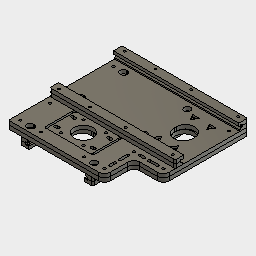
x_carriage humphrito (Autodesk Fusion 360 design; units mm, degrees)
Autodesk Fusion 360 part; units mm, degrees
note: some values were not read from the file. Chosen so that the rebuilt part matches the saved one: how an offset face is resized. Set by a fixed rule: which sketch regions a step uses.
sketch "Sketch1" plane through (0, 0, 0) normal (1, 0, 0) x (0, 0, -1)
  line L0 (0, 0) -> (-127, 0)
  line L1 (-127, 0) -> (-127, 8) construction
  line L2 (-127, 8) -> (0, 8)
  line L3 (0, 8) -> (0, 0)
  line L4 (-127, 4) -> (-123, 0)
  line L5 (-4, 0) -> (0, 4)
  line L6 (-139.5, 14) -> (-121.5, 14)
  line L7 (-121.5, 14) -> (-121.5, -2) construction
  line L8 (-121.5, -2) -> (-139.5, -2)
  line L9 (-139.5, -2) -> (-139.5, 14)
  line L10 (-139.5, 6) -> (-121.5, 6) construction
  line L11 (-128.5, 8.5) -> (-125.5, 8.5)
  line L12 (-125.5, 8.5) -> (-125.5, 3.4142) construction
  line L13 (-125.5, 3.4142) -> (-128.5, 3.4142) construction
  line L14 (-128.5, 3.4142) -> (-128.5, 8.5)
  line L15 (-126.4142, 3.4142) -> (-123.5858, 0.5858)
  line L16 (-125.5, 8.5) -> (-125.5, 8)
  line L17 (-128.5, 3.4142) -> (-126.4142, 3.4142)
  line L18 (-123.5858, 0.5858) -> (-123.5858, -2)
  line L19 (-121.5, 14) -> (-121.5, 8)
  line L20 (-128.5, 6) -> (-139.5, 6)
  line L21 (-127, 4) -> (-127, 8)
  line L22 (-134, 14) -> (-134, -2) construction
  line L23 (-63.5, 8) -> (-63.5, 0) construction
  line L24 (12.5, -2) -> (12.5, 14)
  line L25 (12.5, 14) -> (-5.5, 14)
  line L26 (-5.5, 14) -> (-5.5, -2) construction
  line L27 (-5.5, -2) -> (12.5, -2)
  line L28 (-139.5, -2) -> (12.5, -2)
  line L29 (12.5, -2) -> (12.5, -10)
  line L30 (12.5, -10) -> (-139.5, -10)
  line L31 (-139.5, -10) -> (-139.5, -2)
  line L32 (-76.5, 0) -> (-52, 0)
  line L33 (-52, 0) -> (-52, 4)
  line L34 (-52, 4) -> (-76.5, 4)
  line L35 (-76.5, 4) -> (-76.5, 0)
  line L36 (12.5, -10) -> (-139.5, -10)
  line L37 (-201.5, -18) -> (12.5, -18)
  line L38 (12.5, -18) -> (12.5, -10)
  line L39 (-201.5, -10) -> (-139.5, -10)
  line L40 (-139.5, -10) -> (-139.5, -2)
  line L41 (-139.5, -2) -> (-201.5, -2)
  line L42 (-201.5, -2) -> (-201.5, -10)
  line L43 (-139.5, -10) -> (-201.5, -10)
  line L44 (-201.5, -10) -> (-201.5, -18)
  point P0 (-125, 2)
  dimension "d3" = 8
  dimension "d4" = 127
  dimension "d5" = 45
  dimension "d6" = 4
  dimension "d7" = 45
  dimension "d8" = 4
  dimension "d9" = 18
  dimension "d10" = 4
  dimension "d11" = 3
  dimension "d12" = 0.5
  dimension "d13" = 1.5
  dimension "d14" = 4
  dimension "d15" = 8
  dimension "d16" = 11
  dimension "d17" = 6
  dimension "d19" = 12.5
  dimension "d20" = 8
  dimension "d21" = 4
  dimension "d22" = 24.5
  dimension "d23" = 75
  dimension "d24" = 8
  dimension "d26" = 62
  dimension "d28" = 8
  dimension "d55" = 87.5
  dimension "d230" = 0
  dimension "d231" = 0
  dimension "d232" = 0
  dimension "d233" = 0
  dimension "d252" = 0
  dimension "d253" = 0
  dimension "d254" = 0
  dimension "d255" = 0
  measures "d3" distance of L0.start L2.end
  measures "d4" distance of L1.end L2.end
  measures "d5" angle of L0 L5
  measures "d6" distance of L5.start L5.end
  measures "d7" angle of L0 L4
  measures "d8" distance of L1.end L4.start
  measures "d9" distance of L6.start L6.end
  measures "d10" distance of L7 L12
  measures "d11" distance of L11.start L11.end
  measures "d12" distance of L2 L11
  measures "d13" distance of L1 L14
  measures "d14" distance of L15.start L15.end
  measures "d15" distance of L6 L10
  measures "d16" distance of L9 L14
  measures "d17" distance of L2 L6
  measures "d19" distance of L9 L21
  measures "d20" distance of L24.start L29.end
  measures "d21" distance of L32.start L34.end
  measures "d22" distance of L33.end L34.end
  measures "d23" distance of L21 L33
  measures "d24" distance of L30.end L37.start
  measures "d26" distance of L8.end L41.end
  measures "d28" distance of L39.start L41.end
  measures "d55" distance of L9 L33.end
sketch "Sketch2" plane through (0, 0, 0) normal (0, 1, 0) x (1, 0, 0)
  line L0 (0, -139.5) -> (0, 12.5) construction
  line L1 (0, 12.5) -> (214, 12.5)
  line L2 (214, -139.5) -> (0, -139.5) construction
  line L3 (0, -139.5) -> (0, 12.5)
  line L4 (0, 12.5) -> (152, 12.5)
  line L5 (152, 12.5) -> (152, -201.5) construction
  line L6 (0, -76.5) -> (214, -76.5) construction
  line L7 (214, -76.5) -> (214, -52)
  line L8 (214, -52) -> (0, -52) construction
  line L9 (0, -52) -> (0, -76.5)
  line L10 (152, -64.25) -> (214, -64.25) construction
  line L11 (64.5, -201.5) -> (89, -201.5)
  line L12 (89, -201.5) -> (89, 12.5) construction
  line L13 (89, 12.5) -> (64.5, 12.5)
  line L14 (64.5, 12.5) -> (64.5, -201.5) construction
  line L15 (0, -76.5) -> (0, -52)
  line L16 (0, -76.5) -> (0, -52)
  line L17 (76.75, -201.5) -> (76.75, -139.5) construction
  line L18 (29.75, -139.5) -> (123.75, -139.5)
  line L19 (123.75, -139.5) -> (123.75, -201.5)
  line L20 (123.75, -201.5) -> (29.75, -201.5)
  line L21 (29.75, -201.5) -> (29.75, -139.5)
  circle A0 centre (76.75, -170.5) radius 19.5
  line L22 (123.75, -201.5) -> (29.75, -139.5) construction
  circle A1 centre (53.18, -194.07) radius 2.5
  line L23 (53.18, -194.07) -> (100.32, -194.07) construction
  line L24 (100.32, -194.07) -> (100.32, -146.93) construction
  line L25 (100.32, -146.93) -> (53.18, -146.93) construction
  line L26 (53.18, -146.93) -> (53.18, -194.07) construction
  circle A2 centre (100.32, -194.07) radius 2.5
  circle A3 centre (100.32, -146.93) radius 2.5
  circle A4 centre (53.18, -146.93) radius 2.5
  line L27 (53.18, -194.07) -> (100.32, -146.93) construction
  line L28 (79, -151) -> (74.5, -151)
  arc A5 (74.5, -151) -> (74.5, -190) centre (74.5, -170.5) ccw
  line L29 (74.5, -190) -> (79, -190)
  arc A6 (79, -190) -> (79, -151) centre (79, -170.5) ccw
  line L30 (79, -170.5) -> (74.5, -170.5) construction
  line L31 (0, -201.5) -> (152, -201.5)
  line L32 (214, 12.5) -> (214, -139.5)
  line L33 (53.18, -194.07) -> (29.75, -194.07) construction
  line L34 (0, -139.5) -> (0, -201.5)
  line L35 (0, -201.5) -> (0, 12.5)
  line L36 (0, 0) -> (0, -127)
  line L37 (0, -52) -> (0, -139.5)
  line L38 (0, -139.5) -> (0, -52)
  line L39 (152, -201.5) -> (64.5, -201.5)
  line L40 (0, 12.5) -> (-25, 12.5)
  line L41 (-25, 12.5) -> (-25, -201.5)
  line L42 (-25, -201.5) -> (0, -201.5) construction
  line L43 (0, -201.5) -> (0, 12.5) construction
  line L44 (0, -201.5) -> (152, -201.5) construction
  line L45 (214, -139.5) -> (152, -139.5)
  line L46 (152, -139.5) -> (152, -201.5)
  line L47 (152, -201.5) -> (214, -201.5)
  line L48 (214, -201.5) -> (214, -139.5)
  line L49 (0, -5.5) -> (214, -5.5) construction
  line L50 (0, -121.5) -> (214, -121.5) construction
  line L51 (18, 12.5) -> (18, -201.5) construction
  line L52 (214, 12.5) -> (214, -5.5)
  line L53 (134, 12.5) -> (134, -201.5) construction
  circle A7 centre (183, -64.25) radius 19.5 construction
  line L54 (18, -201.5) -> (0, -201.5)
  line L55 (18, 30.7845) -> (134, 30.7845)
  line L56 (76, 30.7845) -> (76, 24.5879) construction
  line L57 (38.75, -188) -> (114.75, -188) construction
  line L58 (114.75, -188) -> (114.75, -153) construction
  line L59 (114.75, -153) -> (38.75, -153) construction
  line L60 (38.75, -153) -> (38.75, -188) construction
  line L61 (38.75, -188) -> (114.75, -153) construction
  line L62 (114.75, -188) -> (38.75, -153) construction
  circle A8 centre (38.75, -153) radius 2.5
  circle A9 centre (38.75, -188) radius 2.5
  circle A10 centre (114.75, -153) radius 2.5
  circle A11 centre (114.75, -188) radius 2.5
  line L63 (34.75, -159.9282) -> (46.75, -153)
  line L64 (46.75, -153) -> (34.75, -146.0718)
  line L65 (34.75, -146.0718) -> (34.75, -159.9282)
  line L66 (38.75, -148.3812) -> (34.75, -150.6906) construction
  line L67 (34.75, -150.6906) -> (34.75, -155.3094)
  line L68 (34.75, -155.3094) -> (38.75, -157.6188) construction
  line L69 (38.75, -157.6188) -> (42.75, -155.3094)
  line L70 (42.75, -155.3094) -> (42.75, -150.6906) construction
  line L71 (42.75, -150.6906) -> (38.75, -148.3812)
  line L72 (34.75, -181.0718) -> (34.75, -194.9282)
  line L73 (34.75, -194.9282) -> (46.75, -188)
  line L74 (46.75, -188) -> (34.75, -181.0718)
  line L75 (118.75, -159.9282) -> (106.75, -153)
  line L76 (118.75, -146.0718) -> (118.75, -159.9282)
  line L77 (106.75, -153) -> (118.75, -146.0718)
  line L78 (106.75, -188) -> (118.75, -181.0718)
  line L79 (118.75, -181.0718) -> (118.75, -194.9282)
  line L80 (118.75, -194.9282) -> (106.75, -188)
  line L81 (214, -201.5) -> (-25, -201.5)
  line L82 (-25, -201.5) -> (-25, -226.5)
  line L83 (-25, -226.5) -> (214, -226.5)
  line L84 (214, -226.5) -> (214, -201.5)
  line L85 (214, 12.5) -> (239, 12.5)
  line L86 (239, 12.5) -> (239, -226.5)
  line L87 (239, -226.5) -> (214, -226.5)
  line L88 (214, -226.5) -> (214, 12.5)
  line L89 (0, -201.5) -> (0, -226.5)
  circle A12 centre (38.75, -153) radius 6.25
  line L90 (48.75, -142.5) -> (104.75, -142.5) construction
  line L91 (104.75, -142.5) -> (104.75, -198.5) construction
  line L92 (104.75, -198.5) -> (48.75, -198.5) construction
  line L93 (48.75, -198.5) -> (48.75, -142.5) construction
  line L94 (48.75, -142.5) -> (104.75, -198.5) construction
  line L95 (104.75, -142.5) -> (48.75, -198.5) construction
  point P0 (0, -201.5)
  point P1 (0, -139.5)
  point P2 (0, -52)
  point P3 (0, -76.5)
  point P4 (76.75, -170.5)
  point P5 (53.18, -194.07)
  point P6 (0, -201.5)
  point P7 (0, -121.5)
  point P8 (0, -5.5)
  point P9 (183, -64.25)
  point P10 (76.75, -170.5)
  point P11 (38.75, -153)
  point P12 (38.75, -153)
  point P13 (38.75, -188)
  point P14 (76.75, -170.5)
  dimension "d34" = 94
  dimension "d36" = 39
  dimension "d37" = 5
  dimension "d38" = 47.14
  dimension "d39" = 4.5
  dimension "d40" = 19.5
  dimension "d56" = 25
  dimension "d63" = 18
  dimension "d112" = 18
  dimension "d209" = 18
  dimension "d272" = 35
  dimension "d273" = 76
  dimension "d274" = 5
  dimension "d275" = 8
  dimension "d282" = 25
  dimension "d283" = 25
  dimension "d298" = 12.5
  dimension "d299" = 56
  measures "d34" distance of L19.end L20.end
  measures "d36" diameter of A0
  measures "d37" diameter of A1
  measures "d38" distance of P5 L23.end
  measures "d39" distance of A6.centre A5.centre
  measures "d40" radius of A6
  measures "d56" distance of L0.end L40.end
  measures "d63" distance of L1 L49
  measures "d112" distance of L35 L51
  measures "d209" distance of L5 L53
  measures "d272" distance of L57.end L58.end
  measures "d273" distance of L58.end P12
  measures "d274" diameter of A8
  measures "d275" distance of L68 L71
  measures "d282" distance of L41.end L82.end
  measures "d283" distance of L83.end L86.end
  measures "d298" diameter of A12
  measures "d299" distance of L90.start L90.end
sketch "Sketch3" plane through (0, 0, 0) normal (0, 1, 0) x (1, 0, 0)
  line L0 (-25, 12.5) -> (-25, -201.5)
  line L1 (0, -5.5) -> (214, -5.5)
  line L2 (0, 12.5) -> (214, 12.5)
  line L3 (0, 12.5) -> (-25, 12.5)
  line L4 (0, -5.5) -> (-25, -5.5)
  line L5 (214, 12.5) -> (214, -5.5)
  line L6 (239, 5.5) -> (-25, 5.5) construction
  circle A0 centre (-12.5, 5.5) radius 2.25
  circle A1 centre (-12.5, 5.5) radius 2.5
  line L7 (-9.75, 4.5) -> (-9.75, 6.5)
  arc A2 (-9.75, 6.5) -> (-15.25, 6.5) centre (-12.5, 6.5) ccw
  line L8 (-15.25, 6.5) -> (-15.25, 4.5)
  arc A3 (-15.25, 4.5) -> (-9.75, 4.5) centre (-12.5, 4.5) ccw
  line L9 (-12.5, 4.5) -> (-12.5, 6.5) construction
  circle A4 centre (-12.5, 5.5) radius 6.25 construction
  line L10 (107, 5.5) -> (107, 12.5) construction
  circle A5 centre (226.5, 5.5) radius 2.5
  circle A6 centre (226.5, 5.5) radius 2.25
  circle A7 centre (226.5, 5.5) radius 6.25 construction
  line L11 (223.75, 4.5) -> (223.75, 6.5)
  arc A8 (223.75, 4.5) -> (229.25, 4.5) centre (226.5, 4.5) ccw
  line L12 (226.5, 4.5) -> (226.5, 6.5) construction
  line L13 (229.25, 6.5) -> (229.25, 4.5)
  arc A9 (229.25, 6.5) -> (223.75, 6.5) centre (226.5, 6.5) ccw
  circle A10 centre (52.5, 5.5) radius 2.25
  arc A11 (55.25, 6.5) -> (49.75, 6.5) centre (52.5, 6.5) ccw
  arc A12 (49.75, 4.5) -> (55.25, 4.5) centre (52.5, 4.5) ccw
  circle A13 centre (52.5, 5.5) radius 2.5
  line L14 (52.5, 4.5) -> (52.5, 6.5) construction
  line L15 (55.25, 4.5) -> (55.25, 6.5)
  circle A14 centre (52.5, 5.5) radius 6.25 construction
  line L16 (49.75, 6.5) -> (49.75, 4.5)
  circle A15 centre (127.5, 5.5) radius 2.25
  arc A16 (124.75, 4.5) -> (130.25, 4.5) centre (127.5, 4.5) ccw
  circle A17 centre (127.5, 5.5) radius 2.5
  line L17 (124.75, 6.5) -> (124.75, 4.5)
  arc A18 (130.25, 6.5) -> (124.75, 6.5) centre (127.5, 6.5) ccw
  line L18 (127.5, 4.5) -> (127.5, 6.5) construction
  line L19 (130.25, 4.5) -> (130.25, 6.5)
  circle A19 centre (127.5, 5.5) radius 6.25 construction
  line L20 (-41.6156, -63.5) -> (240.5702, -63.5) construction
  line L21 (240.5702, -5.5) -> (240.5702, -121.5) construction
  line L22 (0, -121.5) -> (214, -121.5)
  circle A20 centre (-12.5, -132.5) radius 2.5
  circle A21 centre (52.5, -132.5) radius 2.5
  circle A22 centre (127.5, -132.5) radius 2.5
  circle A23 centre (226.5, -132.5) radius 2.5
  circle A24 centre (-12.5, -132.5) radius 2.25
  circle A25 centre (52.5, -132.5) radius 2.25
  circle A26 centre (127.5, -132.5) radius 2.25
  circle A27 centre (226.5, -132.5) radius 2.25
  line L23 (-12.5, 4.5) -> (-12.5, 4.3)
  arc A28 (-5.75, 6.5) -> (-19.25, 6.5) centre (-12.5, 6.5) ccw construction
  line L24 (-19.25, 6.5) -> (-19.25, 4.5)
  arc A29 (-19.25, 4.5) -> (-5.75, 4.5) centre (-12.5, 4.5) ccw
  line L25 (-5.75, 4.5) -> (-5.75, 6.5)
  line L26 (-19.25, 12.5) -> (-5.75, 12.5)
  line L27 (-5.75, 12.5) -> (-5.75, 6.5)
  line L28 (-5.75, 6.5) -> (-19.25, 6.5) construction
  line L29 (-19.25, 6.5) -> (-19.25, 12.5)
  arc A30 (59.25, 6.5) -> (45.75, 6.5) centre (52.5, 6.5) ccw construction
  line L30 (45.75, 6.5) -> (45.75, 4.5)
  arc A31 (45.75, 4.5) -> (59.25, 4.5) centre (52.5, 4.5) ccw
  line L31 (59.25, 4.5) -> (59.25, 6.5)
  arc A32 (134.25, 6.5) -> (120.75, 6.5) centre (127.5, 6.5) ccw construction
  line L32 (120.75, 6.5) -> (120.75, 4.5)
  arc A33 (120.75, 4.5) -> (134.25, 4.5) centre (127.5, 4.5) ccw
  line L33 (134.25, 4.5) -> (134.25, 6.5)
  line L34 (233.25, 6.5) -> (233.25, 4.5)
  arc A34 (219.75, 4.5) -> (233.25, 4.5) centre (226.5, 4.5) ccw
  line L35 (219.75, 4.5) -> (219.75, 6.5)
  arc A35 (233.25, 6.5) -> (219.75, 6.5) centre (226.5, 6.5) ccw construction
  line L36 (219.75, 12.5) -> (233.25, 12.5)
  line L37 (233.25, 12.5) -> (233.25, 6.5)
  line L38 (233.25, 6.5) -> (219.75, 6.5) construction
  line L39 (219.75, 6.5) -> (219.75, 12.5)
  line L40 (120.75, 12.5) -> (134.25, 12.5)
  line L41 (134.25, 12.5) -> (134.25, 6.5)
  line L42 (134.25, 6.5) -> (120.75, 6.5) construction
  line L43 (120.75, 6.5) -> (120.75, 12.5)
  line L44 (45.75, 12.5) -> (59.25, 12.5)
  line L45 (59.25, 12.5) -> (59.25, 6.5)
  line L46 (59.25, 6.5) -> (45.75, 6.5) construction
  line L47 (45.75, 6.5) -> (45.75, 12.5)
  circle A36 centre (-12.5, -132.5) radius 6.75
  circle A37 centre (52.5, -132.5) radius 6.75
  circle A38 centre (127.5, -132.5) radius 6.75
  circle A39 centre (226.5, -132.5) radius 6.75
  line L48 (239, 12.5) -> (239, -226.5)
  point P0 (-12.5, 5.5)
  point P1 (226.5, 5.5)
  point P2 (52.5, 5.5)
  point P3 (127.5, 5.5)
  dimension "d84" = 4.5
  dimension "d85" = 5
  dimension "d86" = 2.75
  dimension "d87" = 2
  dimension "d88" = 12.5
  dimension "d89" = 12.5
  dimension "d92" = -65
  dimension "d93" = 0
  dimension "d96" = -140
  dimension "d97" = 0
  dimension "d98" = 55
  dimension "d99" = 85
  dimension "d100" = 74
  dimension "d199" = 7
  dimension "d202" = 4.5
  dimension "d242" = 0.2
  dimension "d243" = 4
  dimension "d244" = 6.75
  dimension "d245" = 4
  dimension "d246" = 4
  dimension "d247" = 4
  dimension "d271" = 13.5
  dimension "d284" = 12.5
  measures "d84" diameter of A0
  measures "d85" diameter of A1
  measures "d86" radius of A2
  measures "d87" distance of A3.centre A2.centre
  measures "d88" distance of L0 P0
  measures "d89" diameter of A4
  measures "d199" distance of L2.end L6
  measures "d202" diameter of A24
  measures "d242" distance of A3.centre L23.end
  measures "d244" radius of A29
  measures "d271" diameter of A36
  measures "d284" distance of P1 L48
sketch "Sketch4" plane through (0, 0, 0) normal (0, 1, 0) x (1, 0, 0)
  line L0 (0, 12.5) -> (-25, 12.5) construction
  line L1 (-12.5, 12.5) -> (-12.5, -201.5) construction
  line L2 (-25, -214) -> (214, -214) construction
  line L3 (214, -201.5) -> (214, -139.5) construction
  circle A0 centre (-12.5, -18) radius 2.5
  circle A1 centre (-12.5, -214) radius 2.5
  circle A2 centre (164.5, -214) radius 2.5
  line L4 (164.5, -214) -> (164.5, 12.5) construction
  line L5 (0, 12.5) -> (164.5, 12.5) construction
  line L6 (-12.5, 12.5) -> (0, 12.5) construction
  line L7 (0, -5.5) -> (-25, -5.5) construction
  line L8 (-12.5, -18) -> (14.3422, -18) construction
  line L9 (0, -5.5) -> (164.5, -5.5) construction
  line L10 (164.5, -5.5) -> (164.5, -12) construction
  line L11 (14.3422, -18) -> (158.5, -18) construction
  circle A3 centre (-12.5, -109) radius 2.5
  line L12 (-12.5, -109) -> (158.5, -109) construction
  line L13 (0, -121.5) -> (214, -121.5) construction
  line L14 (0, -121.5) -> (-12.5, -121.5) construction
  line L15 (-12.5, -121.5) -> (-12.5, -109) construction
  line L16 (214, -111.25) -> (152, -111.25)
  line L17 (152, -111.25) -> (152, -17.25)
  line L18 (152, -17.25) -> (214, -17.25)
  line L19 (214, -17.25) -> (214, -111.25)
  line L20 (214, -111.25) -> (152, -17.25) construction
  line L21 (152, -111.25) -> (214, -17.25) construction
  line L22 (123.75, -139.5) -> (123.75, -201.5) construction
  line L23 (123.75, -201.5) -> (29.75, -201.5) construction
  line L24 (152, -139.5) -> (152, -201.5) construction
  line L25 (214, -139.5) -> (0, -139.5) construction
  line L26 (-25, 12.5) -> (-25, -201.5) construction
  line L27 (0, -139.5) -> (-25, -139.5) construction
  line L28 (-12.5, -121.5) -> (-25, -121.5) construction
  circle A4 centre (-12.5, -152) radius 2.5
  line L29 (-12.5, -152) -> (-12.5, -139.5)
  circle A5 centre (164.5, -152) radius 2.5
  line L30 (-12.5, -152) -> (164.5, -152) construction
  line L31 (0, -5.5) -> (214, -5.5) construction
  circle A6 centre (226.5, -114.25) radius 2.5
  circle A7 centre (226.5, -14.25) radius 2.5
  line L32 (-25, -201.5) -> (0, -201.5) construction
  line L33 (163.5, -62) -> (163.5, -66.5)
  arc A8 (163.5, -66.5) -> (202.5, -66.5) centre (183, -66.5) ccw
  line L34 (202.5, -66.5) -> (202.5, -62)
  arc A9 (202.5, -62) -> (163.5, -62) centre (183, -62) ccw
  line L35 (183, -62) -> (183, -66.5) construction
  circle A10 centre (226.5, -14.25) radius 6.25 construction
  circle A11 centre (226.5, -114.25) radius 6.25 construction
  line L36 (226.5, -114.25) -> (226.5, -14.25) construction
  line L37 (183, -64.25) -> (226.5, -64.25) construction
  line L38 (239, 12.5) -> (239, -226.5)
  line L39 (214, -5.5) -> (239, -5.5) construction
  line L40 (226.5, -5.5) -> (226.5, -14.25) construction
  line L41 (214, -201.5) -> (-25, -201.5)
  circle A12 centre (30.5, -214) radius 2.5
  circle A13 centre (121.5, -214) radius 2.5
  line L42 (18, 12.5) -> (18, -201.5)
  line L43 (134, 12.5) -> (134, -201.5)
  line L44 (164.5, -152) -> (167, -152)
  line L45 (164.5, -152) -> (226.5, -152) construction
  circle A14 centre (226.5, -152) radius 2.5
  line L46 (226.5, -152) -> (226.5, -114.25) construction
  point P0 (183, -64.25)
  point P1 (183, -64.25)
  point P2 (214, -201.5)
  point P3 (183, -64.25)
  dimension "d101" = 5
  dimension "d102" = 105
  dimension "d103" = 91
  dimension "d104" = 12.5
  dimension "d105" = 12.5
  dimension "d117" = 19.5
  dimension "d118" = 4.5
  dimension "d213" = 12.5
  dimension "d327" = 100
  dimension "d355" = 12.5
  dimension "d356" = 12.5
  dimension "d357" = 12.5
  measures "d101" diameter of A1
  measures "d102" distance of A1.centre A3.centre
  measures "d103" distance of A0.centre A3.centre
  measures "d104" distance of L7 A0.centre
  measures "d105" distance of A2.centre L24
  measures "d117" radius of A8
  measures "d118" distance of A9.centre A8.centre
  measures "d213" diameter of A10
  measures "d327" distance of A6.centre A7.centre
  measures "d355" distance of A1.centre L41
  measures "d356" distance of A12.centre L42
  measures "d357" distance of A13.centre L43
sketch "Sketch6" plane through (0, 0, 0) normal (0, 1, 0) x (1, 0, 0)
  line L0 (-25, 12.5) -> (239, 12.5)
  line L1 (239, 12.5) -> (239, -226.5)
  line L2 (239, -226.5) -> (-25, -226.5)
  line L3 (-25, -226.5) -> (-25, 12.5)
  point P0 (-25, 12.5)
  point P1 (214, -201.5)
  point P2 (239, -226.5)
extrude "Extrude2" add sketch "Sketch6" against normal up to surface (8 mm away) from surface at -2 makes body 1
extrude "Extrude3" cut sketch "Sketch2" sketch "Sketch4" along normal up to surface contours A0 | A0 L28 L29 A6 | A0 L28 A5 L29 of sketch 2 contours L33 A8 L34 A9 start surface through (0, -2, -12.5) normal (0, 1, 0) end surface through (0, -10, -12.5) normal (0, 1, 0) offset 0 bodies 1
extrude "Extrude4" cut sketch "Sketch4" against normal up to surface (8 mm away) from surface at -2 contours A0 | A1 | A2 | A3 | A4 | A5 | A6 | A7 | A12 | A13 | A14 bodies 1
extrude "Extrude5" cut sketch "Sketch3" against normal up to surface (8 mm away) from surface at -2 contours A0 | A1 | L7 A2 L8 A3 | A5 | A6 | L11 A8 L13 A9 | A10 | A11 A12 L15 L16 | A13 | A15 | A16 L17 A18 L19 | A17 bodies 1
extrude "Extrude6" cut sketch "Sketch3" against normal up to surface (8 mm away) from surface at -2 contours A20 | A21 | A22 | A23 | A24 | A25 | A26 | A27 bodies 1
sketch "Sketch8" plane through (0, 0, 0) normal (0, 1, 0) x (1, 0, 0)
  line L0 (18, 12.5) -> (18, -201.5) construction
  line L1 (0, -201.5) -> (0, 12.5) construction
  line L2 (134, 12.5) -> (134, -201.5) construction
  line L3 (0, -201.5) -> (18, -201.5) construction
  line L4 (18, -201.5) -> (134, -201.5) construction
  line L5 (76, -201.5) -> (76, -159.0464) construction
  circle A0 centre (9, -214) radius 6.5 construction
  line L6 (9, -201.5) -> (9, -214) construction
  circle A1 centre (9, -214) radius 2.5
  circle A2 centre (9, -214) radius 2.25
  line L7 (8, -216.75) -> (10, -216.75)
  arc A3 (10, -216.75) -> (10, -211.25) centre (10, -214) ccw
  line L8 (10, -211.25) -> (8, -211.25)
  arc A4 (8, -211.25) -> (8, -216.75) centre (8, -214) ccw
  line L9 (8, -214) -> (10, -214) construction
  arc A5 (8, -106.25) -> (8, -111.75) centre (8, -109) ccw
  arc A6 (10, -111.75) -> (10, -106.25) centre (10, -109) ccw
  line L10 (8, -109) -> (10, -109) construction
  line L11 (10, -106.25) -> (8, -106.25)
  circle A7 centre (9, -109) radius 6.5 construction
  line L12 (8, -111.75) -> (10, -111.75)
  circle A8 centre (9, -109) radius 2.25
  circle A9 centre (9, -109) radius 2.5
  line L13 (9, -214) -> (9, -109) construction
  line L14 (9, -109) -> (9, -18) construction
  arc A10 (8, -15.25) -> (8, -20.75) centre (8, -18) ccw
  arc A11 (10, -20.75) -> (10, -15.25) centre (10, -18) ccw
  line L15 (8, -18) -> (10, -18) construction
  line L16 (10, -15.25) -> (8, -15.25)
  circle A12 centre (9, -18) radius 6.25 construction
  line L17 (8, -20.75) -> (10, -20.75)
  circle A13 centre (9, -18) radius 2.25
  circle A14 centre (9, -18) radius 2.5
  line L18 (0, -121.5) -> (214, -121.5)
  line L19 (0, -5.5) -> (164.5, -5.5) construction
  circle A15 centre (143, -214) radius 2.5
  circle A16 centre (143, -109) radius 2.5
  circle A17 centre (143, -18) radius 2.5
  circle A18 centre (143, -18) radius 2.25
  circle A19 centre (143, -109) radius 2.25
  circle A20 centre (143, -214) radius 2.25
  arc A21 (8, -11.25) -> (8, -24.75) centre (8, -18) ccw
  line L20 (8, -24.75) -> (10, -24.75)
  arc A22 (10, -24.75) -> (10, -11.25) centre (10, -18) ccw
  line L21 (10, -11.25) -> (8, -11.25)
  arc A23 (8, -102.25) -> (8, -115.75) centre (8, -109) ccw
  line L22 (8, -115.75) -> (10, -115.75)
  arc A24 (10, -115.75) -> (10, -102.25) centre (10, -109) ccw
  line L23 (10, -102.25) -> (8, -102.25)
  arc A25 (8, -207.25) -> (8, -220.75) centre (8, -214) ccw
  line L24 (8, -220.75) -> (10, -220.75)
  arc A26 (10, -220.75) -> (10, -207.25) centre (10, -214) ccw
  line L25 (10, -207.25) -> (8, -207.25)
  circle A27 centre (143, -18) radius 6.75
  circle A28 centre (143, -109) radius 6.75
  circle A29 centre (143, -214) radius 6.75
  line L26 (-25, -226.5) -> (214, -226.5)
  point P0 (9, -214)
  point P1 (9, -109)
  point P2 (9, -109)
  point P3 (9, -18)
  point P4 (9, -18)
  dimension "d129" = 13
  dimension "d131" = 5
  dimension "d132" = 4.5
  dimension "d133" = 2.75
  dimension "d134" = 2
  dimension "d135" = 13
  dimension "d136" = 5
  dimension "d137" = 4.5
  dimension "d138" = 2.75
  dimension "d139" = 2
  dimension "d140" = 12.5
  dimension "d141" = 5
  dimension "d142" = 4.5
  dimension "d143" = 2.75
  dimension "d144" = 2
  dimension "d146" = 12.5
  dimension "d148" = 171
  dimension "d212" = 4.5
  dimension "d264" = 4
  dimension "d265" = 4
  dimension "d266" = 4
  dimension "d267" = 13.5
  dimension "d285" = 12.5
  dimension "d286" = 12.5
  measures "d129" diameter of A0
  measures "d131" diameter of A1
  measures "d132" diameter of A2
  measures "d133" radius of A3
  measures "d134" distance of A4.centre A3.centre
  measures "d135" diameter of A7
  measures "d136" diameter of A9
  measures "d137" diameter of A8
  measures "d138" radius of A6
  measures "d139" distance of A5.centre A6.centre
  measures "d140" diameter of A12
  measures "d141" diameter of A14
  measures "d142" diameter of A13
  measures "d143" radius of A11
  measures "d144" distance of A10.centre A11.centre
  measures "d146" distance of P4 L19
  measures "d212" diameter of A20
  measures "d267" diameter of A27
  measures "d285" distance of P0 L26
  measures "d286" distance of P2 L18
extrude "Extrude7" cut sketch "Sketch8" against normal up to surface (8 mm away) from surface at -2 contours A1 | A2 | L7 A3 L8 A4 | A5 A6 L11 L12 | A8 | A9 | A10 A11 L16 L17 | A13 | A14 | A15 | A16 | A17 | A18 | A19 | A20 bodies 1
extrude "Extrude8" add sketch "Sketch1" along normal up to surface (264 mm away) from surface at -25 separate body contours L4 L8 L9 L14 L15 L17 L18 L20 L28 makes body 2
extrude "Extrude9" add sketch "Sketch1" along normal up to surface (264 mm away) from surface at -25 separate body contours L2 L6 L9 L11 L14 L16 L19 L20 makes body 3
ref_plane "WorkPlane1" through (107, -6, 63.5) normal (0, 0, -1) x (1, 0, 0)
mirror "Mirror1" about plane through (107, -6, 63.5) normal (0, 0, -1) of bodies 2 3 makes body 4 at (151, -2, -1.8905) makes body 5 at (63, 14, -6.5)
copy_body "CopyPasteBodies2" bodies 1 makes body 6
move_body "Move3" bodies 6 to x (1, 0, 0) y (0, 1, 0) z (0, 0, 1) at (0, -8, 0)
copy_body "CopyPasteBodies1" bodies 2 3 makes body 7 makes body 8
move_body "Move1" bodies 7 8 to x (0, 0, -1) y (0, -1, 0) z (-1, 0, 0) at (157.2361, -53.9388, 98.5858)
move_body "Move2" bodies 7 8 to x (1, 0, 0) y (0, 1, 0) z (0, 0, 1) at (-17.7361, 33.9388, 127.9142)
move_face "MoveFace1" by (0, 18, -25) 2 faces at (3.6667, -22.4714, 251.5) (3.6667, -29.5, 251.5) on bodies 7 8
ref_plane "WorkPlane2" through (76, 0, -27.6862) normal (-1, 0, 0) x (0, 0, 1)
mirror "Mirror2" about plane through (76, 0, -27.6862) normal (-1, 0, 0) of bodies 8 7 makes body 9 at (146, -34, 146.8333) makes body 10 at (141.3905, -18, 146.8333)
extrude "Extrude10" cut sketch "Sketch3" along normal up to surface (16 mm away) from surface at -10 contours A0 | A1 | A5 | A6 | A10 | A13 | A15 | A17 | A20 | A21 | A22 | A23 | A24 | A25 | A26 | A27 bodies 2 4
extrude "Extrude11" cut sketch "Sketch3" along normal up to surface (8 mm away) from surface at 6 contours A0 | A6 | A10 | A15 | A24 | A25 | A26 | A27 bodies 3 5
extrude "Extrude19" cut sketch "Sketch8" against normal up to surface (8 mm away) from surface at -18 contours A1 | A2 | A8 | A9 | A13 | A14 | A15 | A16 | A17 | A18 | A19 | A20 bodies 7 10
extrude "Extrude20" cut sketch "Sketch8" against normal up to surface (8 mm away) from surface at -26 contours A2 | A8 | A13 | A18 | A19 | A20 bodies 8 9
sketch "Sketch2 (2)" plane through (0, 0, 0) normal (0, 1, 0) x (1, 0, 0) in component "Glide_screw"
  circle A0 centre (0, 0) radius 2.5
  line L0 (2.3094, 4) -> (-2.3094, 4)
  line L1 (-2.3094, 4) -> (-4.6188, 0)
  line L2 (-4.6188, 0) -> (-2.3094, -4)
  line L3 (-2.3094, -4) -> (2.3094, -4)
  line L4 (2.3094, -4) -> (4.6188, 0)
  line L5 (4.6188, 0) -> (2.3094, 4)
  circle A1 centre (0, 0) radius 6.25
  circle A2 centre (0, 0) radius 2.7
  dimension "d216" = 5
  dimension "d217" = 8
  dimension "d218" = 12.5
  dimension "d219" = 5.4
  dimension "d226" = 0
  dimension "d227" = 0
  dimension "d228" = 0
  dimension "d229" = 0
  dimension "d248" = 0
  dimension "d249" = 0
  dimension "d250" = 0
  dimension "d251" = 0
  measures "d216" diameter of A0
  measures "d217" distance of L0 L3
  measures "d218" diameter of A1
  measures "d219" diameter of A2
extrude "Extrude1" add sketch "Sketch2 (2)" against normal blind 25 separate body contours A0 makes body 11 in component "Glide_screw"
extrude "Extrude2'" add sketch "Sketch2 (2)" along normal blind 3.6 contours A0 | L0 L1 L2 L3 L4 L5 | A2 bodies 11 in component "Glide_screw"
extrude "Extrude3'" add sketch "Sketch2 (2)" against normal blind 1 separate body contours L0 L1 L2 L3 L4 L5 | A1 makes body 12 in component "Glide_screw"
thread "Thread1" "ISO Metric profile 5.0 M5x0.8 6g" major diameter 4.901 minor diameter 3.9895 pitch 0.8 angle 60 resizes the face on face at (2.4876, -8.3333, 0.2489) on bodies 11 in component "Glide_screw"
sketch "Sketch10" plane through (0, 0, 0) normal (0, 1, 0) x (1, 0, 0)
extrude "Extrude12" cut sketch "Sketch3" against normal up to surface (8 mm away) from surface at -10 contours L3 L24 A29 L25 L26 L27 L29 | L2 L30 A31 L31 L44 L45 L47 | L2 L32 A33 L33 L40 L41 L43 | L34 A34 L35 L36 L37 L39 | A36 | A37 | A38 | A39 bodies 6
extrude "Extrude13" cut sketch "Sketch8" along normal up to surface (8 mm away) from surface at -10 contours A21 L20 A22 L21 | A23 L22 A24 L23 | A25 L24 A26 L25 | A27 | A28 | A29 bodies 1
extrude "Extrude14" cut sketch "Sketch2" against normal up to surface (8 mm away) from surface at -10 contours A8 | A9 | A10 | A11 bodies 6
extrude "Extrude15" cut sketch "Sketch2" along normal blind 4 from surface at -18 contours L63 L64 L65 L67 L69 L71 A12 | L63 L65 A12 | L63 L64 A12 | L64 L65 A12 | L72 L73 L74 | L75 L76 L77 | L78 L79 L80 bodies 6
sketch "Sketch11" plane through (0, 0, 0) normal (0, 1, 0) x (1, 0, 0)
  line L0 (29.75, -201.5) -> (29.75, -139.5) construction
  line L1 (123.75, -139.5) -> (123.75, -201.5) construction
  line L2 (214, -139.5) -> (0, -139.5)
  line L3 (214, -201.5) -> (-25, -201.5)
  line L4 (25.75, -139.5) -> (25.75, -201.5)
  line L5 (127.75, -139.5) -> (127.75, -201.5)
  dimension "d287" = 4
  dimension "d288" = 4
  measures "d287" distance of L0 L4
  measures "d288" distance of L1 L5
extrude "Extrude16" cut sketch "Sketch11" against normal up to surface (8 mm away) from surface at -2 bodies 1
sketch "Sketch12" plane through (0, 0, 0) normal (0, 1, 0) x (1, 0, 0)
  line L0 (41.5, -150.25) -> (36, -150.25)
  arc A0 (36, -150.25) -> (36, -155.75) centre (36, -153) ccw
  line L1 (36, -155.75) -> (41.5, -155.75)
  arc A1 (41.5, -155.75) -> (41.5, -150.25) centre (41.5, -153) ccw
  line L2 (41.5, -153) -> (36, -153) construction
  circle A2 centre (36, -153) radius 6.25 construction
  circle A3 centre (41.5, -153) radius 6.25 construction
  curve K0
  line L3 (76.75, -201.5) -> (76.75, -139.5)
  line L4 (112, -150.25) -> (117.5, -150.25)
  line L5 (117.5, -155.75) -> (112, -155.75)
  arc A4 (117.5, -155.75) -> (117.5, -150.25) centre (117.5, -153) ccw
  arc A5 (112, -150.25) -> (112, -155.75) centre (112, -153) ccw
  arc A6 (41.5, -190.75) -> (41.5, -185.25) centre (41.5, -188) ccw
  line L6 (41.5, -190.75) -> (36, -190.75)
  arc A7 (36, -185.25) -> (36, -190.75) centre (36, -188) ccw
  line L7 (36, -185.25) -> (41.5, -185.25)
  line L8 (112, -190.75) -> (117.5, -190.75)
  arc A8 (117.5, -190.75) -> (117.5, -185.25) centre (117.5, -188) ccw
  arc A9 (112, -185.25) -> (112, -190.75) centre (112, -188) ccw
  line L9 (117.5, -185.25) -> (112, -185.25)
  point P0 (38.75, -153)
  point P1 (114.75, -153)
  point P2 (114.75, -188)
  point P3 (38.75, -188)
  point P4 (38.75, -153)
  dimension "d340" = 5.5
  dimension "d341" = 2.75
  dimension "d342" = 12.5
  measures "d340" distance of A1.centre A0.centre
  measures "d341" radius of A1
  measures "d342" diameter of A3
sketch "Sketch14" plane through (0, 0, 0) normal (0, 1, 0) x (1, 0, 0)
  line L0 (53.18, -194.07) -> (100.32, -194.07)
  line L1 (53.18, -146.93) -> (53.18, -194.07)
  line L2 (50.43, -201.07) -> (55.93, -201.07)
  arc A0 (55.93, -201.07) -> (55.93, -187.07) centre (55.93, -194.07) ccw
  line L3 (55.93, -187.07) -> (50.43, -187.07)
  arc A1 (50.43, -187.07) -> (50.43, -201.07) centre (50.43, -194.07) ccw
  line L4 (50.43, -194.07) -> (55.93, -194.07) construction
  line L5 (58.0198, -197.4823) -> (59.93, -193.9664) construction
  line L6 (59.93, -193.9664) -> (57.8402, -190.5541) construction
  line L7 (57.8402, -190.5541) -> (53.8402, -190.6577) construction
  line L8 (53.8402, -190.6577) -> (51.93, -194.1736) construction
  line L9 (51.93, -194.1736) -> (54.0198, -197.5859) construction
  line L10 (54.0198, -197.5859) -> (58.0198, -197.4823) construction
  circle A2 centre (55.93, -194.07) radius 6.25 construction
  point P0 (53.18, -194.07)
  point P1 (55.93, -194.07)
  dimension "d348" = 7
  dimension "d349" = 4
  dimension "d350" = 5.5
  dimension "d351" = 12.5
  measures "d348" radius of A0
  measures "d349" distance of P1 L5.end
  measures "d350" distance of A1.centre P1
  measures "d351" diameter of A2
extrude "Extrude17" add sketch "Sketch2" along normal up to surface (8 mm away) from surface at -10 separate body contours L11 L18 L19 L20 L21 L31 L39 L81 | A0 L28 L29 A6 | A0 L28 A5 L29 | A8 | A9 | A10 | A11 | L63 L64 L65 L67 L69 L71 A12 | L63 L69 A12 | L63 L65 A12 | L63 L64 A12 | L65 L67 A12 | L64 L65 A12 | L64 L71 A12 | L72 L73 L74 | L75 L76 L77 | L78 L79 L80 makes body 13
extrude "Extrude24" cut sketch "Sketch12" against normal up to surface (8 mm away) from surface at -2 bodies 13
copy_body "Body->Comp4" bodies 13 removing the originals makes body 14 in component "motor_plate"
sketch "Sketch1 (2)" plane through (0, 0, 0) normal (0, 1, 0) x (1, 0, 0) in component "motor_plate"
  line L0 (106.75, -153) -> (118.75, -146.0718)
  line L1 (118.75, -146.0718) -> (118.75, -159.9282)
  line L2 (118.75, -159.9282) -> (106.75, -153)
  circle A0 centre (114.75, -153) radius 2.5
  circle A1 centre (38.75, -153) radius 2.5
  line L3 (46.75, -153) -> (34.75, -146.0718)
  line L4 (34.75, -146.0718) -> (34.75, -159.9282)
  line L5 (34.75, -159.9282) -> (46.75, -153)
  line L6 (46.75, -188) -> (34.75, -181.0718)
  line L7 (34.75, -181.0718) -> (34.75, -194.9282)
  line L8 (34.75, -194.9282) -> (46.75, -188)
  line L9 (106.75, -188) -> (118.75, -181.0718)
  line L10 (118.75, -181.0718) -> (118.75, -194.9282)
  line L11 (118.75, -194.9282) -> (106.75, -188)
  circle A2 centre (114.75, -188) radius 2.5
  circle A3 centre (38.75, -188) radius 2.5
  line L12 (25.75, -139.5) -> (25.75, -201.5)
  line L13 (127.75, -139.5) -> (127.75, -201.5)
  line L14 (214, -139.5) -> (0, -139.5)
  line L15 (214, -201.5) -> (-25, -201.5)
extrude "Extrude21" cut sketch "Sketch1 (2)" against normal up to surface (8 mm away) from surface at -2 contours L0 L1 L2 | A0 | A1 | L3 L4 L5 | L6 L7 L8 | L9 L10 L11 | A2 | A3 | L12 L13 L14 L15 sketch seen with x (0, 0, -1) y (0, -1, 0) z (-1, 0, 0) at (353.5, -20, 141) bodies 6
extrude "Extrude22" cut sketch "Sketch1 (2)" against normal up to surface (8 mm away) from surface at -10 contours A0 | A1 | A2 | A3 sketch seen with x (0, 0, -1) y (0, -1, 0) z (-1, 0, 0) at (353.5, -20, 141) bodies 1
extrude "Extrude23" cut sketch "Sketch1 (2)" along normal blind 4 from surface at -18 contours L0 L1 L2 | L3 L4 L5 | L6 L7 L8 | L9 L10 L11 sketch seen with x (0, 0, -1) y (0, -1, 0) z (-1, 0, 0) at (353.5, -20, 141) bodies 1
sketch "Sketch2 (3)" plane through (0, -10, 0) normal (0, -1, 0) x (1, 0, 0) in component "motor_plate"
  circle A0 centre (53.18, 146.93) radius 2.5
  circle A1 centre (100.32, 146.93) radius 2.5
  circle A2 centre (100.32, 194.07) radius 2.5
  circle A3 centre (76.75, 170.5) radius 19.5 construction
  circle A4 centre (53.18, 194.07) radius 2.5
  line L0 (29.75, 139.5) -> (123.75, 139.5)
  line L1 (123.75, 139.5) -> (123.75, 201.5)
  line L2 (123.75, 201.5) -> (29.75, 201.5) construction
  line L3 (29.75, 201.5) -> (29.75, 139.5)
  line L4 (60.1082, 198.07) -> (46.2518, 198.07)
  line L5 (46.2518, 198.07) -> (53.18, 186.07)
  line L6 (53.18, 186.07) -> (60.1082, 198.07)
  line L7 (53.18, 194.07) -> (100.32, 194.07) construction
  line L8 (100.32, 194.07) -> (100.32, 146.93) construction
  line L9 (53.18, 194.07) -> (53.18, 146.93) construction
  line L10 (53.18, 170.5) -> (100.32, 170.5) construction
  line L11 (76.75, 194.07) -> (76.75, 170.5) construction
  line L12 (46.2518, 142.93) -> (53.18, 154.93)
  line L13 (60.1082, 142.93) -> (46.2518, 142.93)
  line L14 (53.18, 154.93) -> (60.1082, 142.93)
  line L15 (100.32, 186.07) -> (93.3918, 198.07)
  line L16 (93.3918, 198.07) -> (107.2482, 198.07)
  line L17 (107.2482, 198.07) -> (100.32, 186.07)
  line L18 (107.2482, 142.93) -> (100.32, 154.93)
  line L19 (100.32, 154.93) -> (93.3918, 142.93)
  line L20 (93.3918, 142.93) -> (107.2482, 142.93)
  line L21 (53.18, 194.07) -> (53.18, 198.07)
  arc A5 (41.5, 185.25) -> (41.5, 190.75) centre (41.5, 188) ccw
  line L22 (41.5, 185.25) -> (36, 185.25)
  arc A6 (36, 190.75) -> (36, 185.25) centre (36, 188) ccw
  line L23 (36, 190.75) -> (41.5, 190.75)
  line L24 (117.5, 185.25) -> (112, 185.25)
  arc A7 (112, 190.75) -> (112, 185.25) centre (112, 188) ccw
  line L25 (112, 190.75) -> (117.5, 190.75)
  arc A8 (117.5, 185.25) -> (117.5, 190.75) centre (117.5, 188) ccw
  arc A9 (41.5, 150.25) -> (41.5, 155.75) centre (41.5, 153) ccw
  line L26 (41.5, 150.25) -> (36, 150.25)
  arc A10 (36, 155.75) -> (36, 150.25) centre (36, 153) ccw
  line L27 (36, 155.75) -> (41.5, 155.75)
  arc A11 (117.5, 150.25) -> (117.5, 155.75) centre (117.5, 153) ccw
  line L28 (117.5, 150.25) -> (112, 150.25)
  arc A12 (112, 155.75) -> (112, 150.25) centre (112, 153) ccw
  line L29 (112, 155.75) -> (117.5, 155.75)
  point P0 (53.18, 194.07)
  dimension "d328" = 13.8564
  dimension "d331" = 4
  measures "d328" distance of L4.start L4.end
  measures "d331" distance of P0 L21.end
extrude "Extrude1'" cut sketch "Sketch2 (3)" against normal blind 4 contours L4 L5 L6 | L12 L13 L14 | L15 L16 L17 | L18 L19 L20 bodies 14 in component "motor_plate"
fillet "Fillet1" radius 5 4 edges at (29.75, -6, 201.5) (123.75, -6, 201.5) (123.75, -6, 139.5) (29.75, -6, 139.5) on bodies 14 in component "motor_plate"
sketch "Sketch15" plane through (0, 0, 0) normal (0, 1, 0) x (1, 0, 0)
  line L0 (239, -226.5) -> (177, -226.5)
  line L1 (177, -226.5) -> (177, -164.5)
  line L2 (177, -164.5) -> (239, -164.5)
  line L3 (239, -164.5) -> (239, -226.5)
  line L4 (164.5, -214) -> (164.5, 12.5) construction
  line L5 (164.5, -152) -> (226.5, -152) construction
  line L6 (167, -182) -> (167, -164)
  arc A0 (167, -164) -> (162, -164) centre (164.5, -164) ccw
  line L7 (162, -164) -> (162, -182)
  arc A1 (162, -182) -> (167, -182) centre (164.5, -182) ccw
  line L8 (164.5, -182) -> (164.5, -164) construction
  line L9 (196.5, -154.5) -> (214.5, -154.5)
  arc A2 (214.5, -154.5) -> (214.5, -149.5) centre (214.5, -152) ccw
  line L10 (214.5, -149.5) -> (196.5, -149.5)
  arc A3 (196.5, -149.5) -> (196.5, -154.5) centre (196.5, -152) ccw
  line L11 (196.5, -152) -> (214.5, -152) construction
  line L12 (167, -202) -> (167, -192)
  arc A4 (167, -192) -> (162, -192) centre (164.5, -192) ccw
  line L13 (162, -192) -> (162, -202)
  arc A5 (162, -202) -> (167, -202) centre (164.5, -202) ccw
  line L14 (164.5, -202) -> (164.5, -192) construction
  line L15 (176.5, -154.5) -> (186.5, -154.5)
  arc A6 (186.5, -154.5) -> (186.5, -149.5) centre (186.5, -152) ccw
  line L16 (186.5, -149.5) -> (176.5, -149.5)
  arc A7 (176.5, -149.5) -> (176.5, -154.5) centre (176.5, -152) ccw
  line L17 (176.5, -152) -> (186.5, -152) construction
  point P0 (239, -226.5)
  dimension "d359" = 12.5
  dimension "d360" = 12.5
  dimension "d361" = 5
  dimension "d362" = 5
  dimension "d363" = 10
  dimension "d364" = 12
  dimension "d365" = 12
  dimension "d366" = 12
  dimension "d367" = 12
  dimension "d368" = 10
  dimension "d369" = 10
  dimension "d370" = 10
  measures "d359" distance of L1 L4
  measures "d360" distance of L2 L5
  measures "d361" distance of L6 L7
  measures "d362" distance of L9 L10
  measures "d363" distance of A3.centre A6.centre
  measures "d364" distance of L5.end A2.centre
  measures "d365" distance of L5.start A7.centre
  measures "d366" distance of L5.start A0.centre
  measures "d367" distance of L4.start A5.centre
  measures "d368" distance of A1.centre A4.centre
  measures "d369" distance of A5.centre A4.centre
  measures "d370" distance of A7.centre A6.centre
extrude "Extrude26" cut sketch "Sketch15" against normal up to surface (16 mm away) from surface at -2 bodies 1 6
fillet "Fillet1'" radius 12.5 2 edges at (177, -6, 164.5) (177, -14, 164.5) on bodies 1 6
fillet "Fillet2" radius 12.5 4 edges at (177, -6, 226.5) (239, -6, 164.5) (177, -14, 226.5) (239, -14, 164.5) on bodies 1 6
fillet "Fillet3" radius 3 6 edges at (-25, -6, 226.5) (-25, -6, -12.5) (239, -6, -12.5) (-25, -14, 226.5) (-25, -14, -12.5) (239, -14, -12.5) on bodies 1 6
fillet "Fillet4" radius 3 16 edges at (239, 2, 139.5) (-25, 2, 139.5) (239, 10, 139.5) (-25, 10, 139.5) (-25, 2, -12.5) (239, 2, -12.5) (-25, 10, -12.5) (239, 10, -12.5) (0, -22, -12.5) (0, -22, 226.5) (0, -30, -12.5) (0, -30, 226.5) (152, -30, -12.5) (152, -30, 226.5) (152, -22, -12.5) (152, -22, 226.5) on bodies 2 3 4 5 7 8 9 10
fillet "Fillet5" radius 3 8 edges at (127.75, -6, 201.5) (25.75, -6, 201.5) (25.75, -6, 139.5) (127.75, -6, 139.5) (152, -14, 115.25) (214, -14, 115.25) (214, -14, 13.25) (152, -14, 13.25) on bodies 1 6
component "Glide_screw" placed x (1, 0, 0) y (0, -1, 0) z (0, 0, -1) at (-12.5, -11, -4.5)
component "motor_plate" placed x (1, 0, 0) y (0, 1, 0) z (0, 0, 1) at (0, 0, 0)
component "motor_plate" placed x (0, 0, -1) y (0, -1, 0) z (-1, 0, 0) at (353.5, -20, 141)
equation "thinness = 8 mm"
equation "rail_height = 127 mm"
equation "d3 = thinness"
equation "d4 = rail_height"
equation "d20 = thinness"
equation "d24 = thinness"
equation "d28 = thinness"
equation "d36 = ( 19.5 * 2 ) * 1 mm"
equation "d117 = 39 mm / 2"
equation "d209 = d112"
equation "d267 = ( 6.75 * 2 ) * 1 mm"
equation "d282 = d56"
equation "d283 = d56"
equation "d284 = d88"
equation "d288 = d287"
equation "d341 = ( 5.5 / 2 ) * 1 mm"
equation "d356 = d355"
equation "d357 = d355"
equation "d366 = d365"
equation "d367 = d364"
equation "d368 = d363"
named bodies: "X-axis_plate", "Z-axis_plate"
